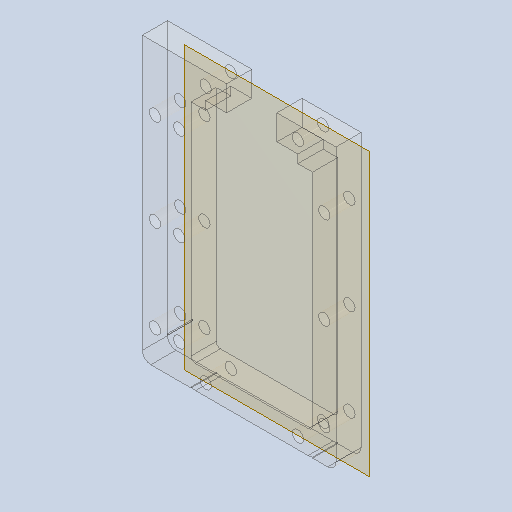
# Autodesk Inventor part: _body_side_ver2
Saved by Autodesk Inventor 2024.3 (Build 283343000, 343)
## iProperties
Created: 2024-09-09
Part Number: _body_side_ver2
Material: PMMA 플라스틱
Document SubType Name: Modeling
Designer: gretc
Density: 1.188 g/cm^3
Appearance: 폴리카보네이트 - 선명
Mass: 9.67014 g
Surface Area: 56.6778 cm^2
Volume: 8.13985 cm^3
Author: gretc
Autodesk Inventor part; units mm, degrees
ref_plane "YZ Plane" through (0, 0, 0) normal (1, 0, 0) x (0, 1, 0)
ref_plane "XZ Plane" through (0, 0, 0) normal (0, 1, 0) x (-1, 0, 0)
ref_plane "XY Plane" through (0, 0, 0) normal (0, 0, 1) x (1, 0, 0)
ref_plane "작업 평면1" through (0, 0, 0) normal (0, 0, 1) x (1, 0, 0)
sketch "스케치1" plane through (0, 0, 0) normal (0, 0, 1) x (1, 0, 0)
  arc A0 (20.1, 4.5766) -> (19.5808, 6.2636) centre (17.1, 4.5766) ccw projected
  line L0 (19.5808, 6.2636) -> (15.5953, 12.1246) projected
  arc A1 (15.5953, 12.1246) -> (13.9414, 13) centre (13.9414, 11) ccw projected
  line L1 (13, 13) -> (13.9414, 13) projected
  arc A2 (14.5, 11.5) -> (13, 13) centre (13, 11.5) ccw projected
  line L2 (14.5, -41.5) -> (14.5, 11.5) projected
  arc A3 (13.5, -42.5) -> (14.5, -41.5) centre (13.5, -41.5) ccw projected
  line L3 (-13.5, -42.5) -> (13.5, -42.5) projected
  arc A4 (-14.5, -41.5) -> (-13.5, -42.5) centre (-13.5, -41.5) ccw projected
  line L4 (-14.5, 11.5) -> (-14.5, -41.5) projected
  arc A5 (-13, 13) -> (-14.5, 11.5) centre (-13, 11.5) ccw projected
  line L5 (-13.9414, 13) -> (-13, 13) projected
  arc A6 (-13.9414, 13) -> (-15.5953, 12.1246) centre (-13.9414, 11) ccw projected
  line L6 (-15.5953, 12.1246) -> (-19.5808, 6.2636) projected
  arc A7 (-19.5808, 6.2636) -> (-20.1, 4.5766) centre (-17.1, 4.5766) ccw projected
  line L7 (-20.1, 4.5766) -> (-20.1, -39.6766) projected
  arc A8 (-20.1, -39.6766) -> (-19.5808, -41.3636) centre (-17.1, -39.6766) ccw projected
  line L8 (-19.5808, -41.3636) -> (-15.8929, -46.7869) projected
  arc A9 (-15.8929, -46.7869) -> (-13.4121, -48.1) centre (-13.4121, -45.1) ccw projected
  line L9 (-13.4121, -48.1) -> (13.4121, -48.1) projected
  arc A10 (13.4121, -48.1) -> (15.8929, -46.7869) centre (13.4121, -45.1) ccw projected
  line L10 (15.8929, -46.7869) -> (19.5808, -41.3636) projected
  arc A11 (19.5808, -41.3636) -> (20.1, -39.6766) centre (17.1, -39.6766) ccw projected
  line L11 (20.1, -39.6766) -> (20.1, 4.5766) projected
  circle A12 centre (-17.3, 4) radius 1.35 projected
  circle A13 centre (-17.3, -18) radius 1.35 projected
  circle A14 centre (-11, -45.3) radius 1.35 projected
  circle A15 centre (17.3, 4) radius 1.35 projected
  circle A16 centre (17.3, -18) radius 1.35 projected
  circle A17 centre (11, -45.3) radius 1.35 projected
  circle A18 centre (-17.3, -40) radius 1.35 projected
  circle A19 centre (17.3, -40) radius 1.35 projected
  line L12 (-20.1, -48.0993) -> (-20.1, 25.0993) projected
  line L13 (-20.1, 25.0993) -> (-26.1, 25.0993) projected
  line L14 (-26.1, -48.0993) -> (-26.1, 25.0993) projected
  line L15 (-20.1, -48.0993) -> (-26.1, -48.0993) projected
  line L16 (-14.5, 11.5) -> (-14.5, 13.7353)
  line L17 (-13.9414, 13) -> (-15.2676, 13)
  line L18 (-14.5, -41.5) -> (-14.5, -54.5935)
  line L19 (-20.1, -48.0993) -> (-13.475, -48.0993)
  line L20 (-13.475, -48.0993) -> (-26.1, -48.0993)
  line L21 (-26.1, -48.0993) -> (-26.1, 13)
  line L22 (-26.1, 13) -> (-13.475, 13)
  line L23 (-13.475, 13) -> (-13.475, -48.0993)
  line L24 (-17.3, 4) -> (-17.3, -18)
  line L25 (-17.3, -18) -> (-23.1, -18)
  line L26 (-23.1, -18) -> (-23.1, 4)
  line L27 (-23.1, 4) -> (-17.3, 4)
  line L28 (-17.3, -18) -> (-17.3, -40)
  line L29 (-17.3, -40) -> (-23.1, -40)
  line L30 (-23.1, -40) -> (-23.1, -18)
  line L31 (-23.1, -18) -> (-17.3, -18)
  circle A20 centre (-23.1, 4) radius 1.35
  circle A21 centre (-23.1, -18) radius 1.35
  circle A22 centre (-23.1, -40) radius 1.35
  line L32 (14.5, 13) -> (14.5, -48.0993)
  line L33 (14.5, -48.0993) -> (20.1, -48.0993)
  line L34 (20.1, -48.0993) -> (20.1, 13)
  line L35 (20.1, 13) -> (14.5, 13)
  circle A23 centre (-23.1, 4) radius 1.35 projected
  circle A24 centre (-23.1, -18) radius 1.35 projected
  circle A25 centre (-23.1, -40) radius 1.35 projected
  point P0 (0, 0)
  point P1 (-14.5, 13)
  point P2 (20.1, 4.5766)
  point P3 (14.5, 11.5)
  point P4 (-26.1, 13)
  point P5 (-14.5, -48.0993)
  point P6 (-14.5, -47.8958)
  point P7 (14.5, -47.8958)
  point P8 (20.1, -39.6766)
  point P9 (-20.0825, -40)
  point P10 (-20.1, -40)
  dimension "d0" = 2.7
  dimension "d1" = 2.7
  dimension "d2" = 2.7
  constraints: 40 end point, 8 parallel, 6 perpendicular, 5 coincident, 4 vertical, 3 centre point, 2 horizontal, 2 point on line, 1 point on circle
  measures "d0" diameter of A20
  measures "d1" diameter of A21
  measures "d2" diameter of A22
extrude "돌출1" add sketch "스케치1" along normal blind 6 contours L11 A11 L10 A10 L32 L2 A1 L0 A0 | A0 L0 A1 L32 L35 L34 | L34 L33 L32 A10 L10 A11 | A10 L9 A9 L23 L3 A3 L32 | L23 A9 L18 A4 L3 | L18 L19 L12 L29 A8 L8 A9 | A9 L8 A8 L29 A18 L28 A13 L24 A12 L27 L7 A7 L6 A6 L16 L4 L18 | L15 L14 L22 L12 L7 L27 A20 L26 A21 L30 A22 L29 | A6 L6 A7 L12 L22 L17 L16 | L29 A22 L30 A21 L25 L7 L12 | A8 L7 L25 A13 L28 A18 L29 | L25 A21 L26 A20 L27 L7 | L7 L27 A12 L24 A13 L25
fillet "모깎기1" radius 2 6 edges at (-26.1, -48.0993, 3) (20.1, -48.0993, 3) (20.1, 13, 3) (14.5, 13, 3) (-14.5, 13, 3) (-26.1, 13, 3)
sketch "스케치2" plane through (0, 0, 6) normal (0, 0, 1) x (1, 0, 0)
  line L0 (-13, 13) -> (-13, 19) projected
  line L1 (13, 13) -> (-13, 13) projected
  line L2 (13, 13) -> (13, 19) projected
  line L3 (-13, 19) -> (13, 19) projected
  arc A0 (-24.1, 13) -> (-26.1, 11) centre (-24.1, 11) ccw projected
  line L4 (-26.1, 11) -> (-26.1, -46.0993) projected
  arc A1 (-26.1, -46.0993) -> (-24.1, -48.0993) centre (-24.1, -46.0993) ccw projected
  line L5 (-24.1, -48.0993) -> (-14.5, -48.0993) projected
  line L6 (-14.5, -48.0993) -> (-14.5, -47.8958) projected
  arc A2 (-14.5, -47.8958) -> (-13.4121, -48.1) centre (-13.4121, -45.1) ccw projected
  line L7 (-13.4121, -48.1) -> (13.4121, -48.1) projected
  arc A3 (13.4121, -48.1) -> (14.5, -47.8958) centre (13.4121, -45.1) ccw projected
  line L8 (14.5, -47.8958) -> (14.5, -48.0993) projected
  line L9 (14.5, -48.0993) -> (18.1, -48.0993) projected
  arc A4 (18.1, -48.0993) -> (20.1, -46.0993) centre (18.1, -46.0993) ccw projected
  line L10 (20.1, -46.0993) -> (20.1, 11) projected
  arc A5 (20.1, 11) -> (18.1, 13) centre (18.1, 11) ccw projected
  line L11 (18.1, 13) -> (16.5, 13) projected
  arc A6 (16.5, 13) -> (14.5, 11) centre (16.5, 11) ccw projected
  line L12 (14.5, 11) -> (14.5, -41.5) projected
  arc A7 (13.5, -42.5) -> (14.5, -41.5) centre (13.5, -41.5) ccw projected
  line L13 (13.5, -42.5) -> (-13.5, -42.5) projected
  arc A8 (-14.5, -41.5) -> (-13.5, -42.5) centre (-13.5, -41.5) ccw projected
  line L14 (-14.5, -41.5) -> (-14.5, 11) projected
  arc A9 (-14.5, 11) -> (-16.5, 13) centre (-16.5, 11) ccw projected
  line L15 (-16.5, 13) -> (-24.1, 13) projected
  circle A10 centre (-17.3, -18) radius 1.35 projected
  circle A11 centre (-23.1, 4) radius 1.35 projected
  circle A12 centre (-23.1, -18) radius 1.35 projected
  circle A13 centre (11, -45.3) radius 1.35 projected
  circle A14 centre (-11, -45.3) radius 1.35 projected
  circle A15 centre (-17.3, 4) radius 1.35 projected
  circle A16 centre (-17.3, -40) radius 1.35 projected
  circle A17 centre (17.3, -18) radius 1.35 projected
  circle A18 centre (17.3, 4) radius 1.35 projected
  circle A19 centre (17.3, -40) radius 1.35 projected
  arc A20 (-20.1, -39.6766) -> (-20.0825, -40) centre (-17.1, -39.6766) ccw projected
  line L16 (-20.0825, -40) -> (-20.1, -40) projected
  line L17 (-20.1, -40) -> (-20.1, -39.6766) projected
  circle A21 centre (-23.1, -40) radius 1.35 projected
  line L18 (18.1, 11) -> (-24.1, 11)
  line L19 (-24.1, 11) -> (-26.1, 11)
  line L20 (18.1, 11) -> (20.1, 11)
  line L21 (20.1, 11) -> (-26.1, 11)
  line L22 (-26.1, 11) -> (-26.1, 19)
  line L23 (-26.1, 19) -> (20.1, 19)
  line L24 (20.1, 19) -> (20.1, 11)
  line L25 (11, -45.3) -> (-11, -45.3)
  line L26 (-11, -45.3) -> (-11, 16)
  line L27 (-11, 16) -> (11, 16)
  line L28 (11, 16) -> (11, -45.3)
  circle A22 centre (11, 16) radius 1.35
  circle A23 centre (-11, 16) radius 1.35
  line L29 (11, 16) -> (6, 16)
  line L30 (-11, 16) -> (-6, 16)
  line L31 (6, 13) -> (6, 19)
  line L32 (6, 19) -> (-6, 19)
  line L33 (-6, 19) -> (-6, 13)
  line L34 (-6, 13) -> (6, 13)
  point P0 (0, 0)
  point P1 (11, 13)
  point P2 (11, 11)
  point P3 (-11, 13)
  point P4 (-14.5, 11)
  point P5 (-11, 11)
  dimension "d6" = 2.7
  dimension "d7" = 2.7
  dimension "d8" = 5
  dimension "d9" = 5
  constraints: 34 end point, 7 equal length, 5 perpendicular, 4 point on line, 3 horizontal, 2 centre point, 2 coincident
  measures "d6" diameter of A22
  measures "d7" diameter of A23
  measures "d8" distance of L29.start L29.end
  measures "d9" distance of L30.start L30.end
extrude "돌출2" add sketch "스케치2" against normal blind 6 contours L1 L26 L18 A9 L15 A0 L22 L23 L0 | L0 L3 L33 L27 A23 L26 L1 | L26 A23 L27 L33 L1 | L3 L2 L1 L28 A22 L27 L31 | L31 L27 A22 L28 L1 | L28 L1 L2 L23 L24 A5 L11 A6 L18
